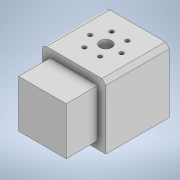
# Autodesk Inventor part: PracticeCube
Saved by Autodesk Inventor 2022 (Build 260153000, 153)
## iProperties
Created: 2021-09-22
Part Number: PracticeCube
Material: Generic
Document SubType Name: Modeling
Designer: merky
Density: 1 g/cm^3
Appearance: Default
Author: merky
Autodesk Inventor part; units mm, degrees
ref_plane "YZ Plane" through (0, 0, 0) normal (1, 0, 0) x (0, 1, 0)
ref_plane "XZ Plane" through (0, 0, 0) normal (0, 1, 0) x (-1, 0, 0)
ref_plane "XY Plane" through (0, 0, 0) normal (0, 0, 1) x (1, 0, 0)
sketch "Sketch1" plane through (0, 0, 0) normal (0, 1, 0) x (-1, 0, 0)
  line L0 (0, 0) -> (-101.6, 0)
  line L1 (-101.6, 0) -> (-101.6, -101.6)
  line L2 (-101.6, -101.6) -> (0, -101.6)
  line L3 (0, -101.6) -> (0, 0)
  dimension "d1" = 101.6
  dimension "d2" = 101.6
  constraints: 8 end point, 2 parallel, 1 horizontal, 1 perpendicular
  measures "d1" distance of L1.end L0.end
  measures "d2" distance of L1.end L2.end
extrude "Extrusion1" add sketch "Sketch1" along normal blind 101.6
sketch "Sketch2" plane through (0, 101.6, 0) normal (0, 1, 0) x (1, 0, 0)
  point P0 (0, 0)
  point P1 (50.8, 50.8)
hole "Hole1" at (50.8, 101.6, -50.8) direction (0, -1, 0) diameter 19.05 end through all
sketch "Sketch3" plane through (0, 101.6, 0) normal (0, 1, 0) x (1, 0, 0)
  point P0 (0, 0)
  point P1 (25.6286, 50.8)
  point P2 (50.8, 50.8)
  point P3 (38.2143, 29.0009)
  point P4 (63.3857, 29.0009)
  point P5 (75.9714, 50.8)
  point P6 (63.3857, 72.5991)
  point P7 (38.2143, 72.5991)
  dimension "d17" = 360
  constraints: 7 other
hole "Hole2" at (25.6286, 101.6, -50.8) at (50.8, 101.6, -50.8) at (38.2143, 101.6, -29.0009) at (63.3857, 101.6, -29.0009) at (75.9714, 101.6, -50.8) at (63.3857, 101.6, -72.5991) at (38.2143, 101.6, -72.5991) direction (0, -1, 0) diameter 6.35 end through all
chamfer "Chamfer1" distance 6.35 angle 45 1 edges at (101.6, 101.6, -50.8)
fillet "Fillet1" radius 6.35 1 edges at (0, 101.6, -50.8)
sketch "Sketch4" plane through (0, 0, 0) normal (0, 0, 1) x (1, 0, 0)
  line L0 (12.7, 88.9) -> (88.9, 88.9)
  line L1 (88.9, 88.9) -> (88.9, 12.7)
  line L2 (88.9, 12.7) -> (12.7, 12.7)
  line L3 (12.7, 12.7) -> (12.7, 88.9)
  line L4 (12.7, 88.9) -> (88.9, 12.7) construction
  line L5 (88.9, 88.9) -> (12.7, 12.7) construction
  point P0 (0, 0)
  point P1 (50.8, 50.8)
  dimension "d30" = 76.2
  dimension "d31" = 76.2
  constraints: 12 end point, 2 midpoint, 2 parallel, 1 horizontal, 1 perpendicular
  measures "d30" distance of L1.end L2.end
  measures "d31" distance of L0.end L1.end
extrude "Extrusion3" add sketch "Sketch4" along normal blind 50.8
body "Solid1"
